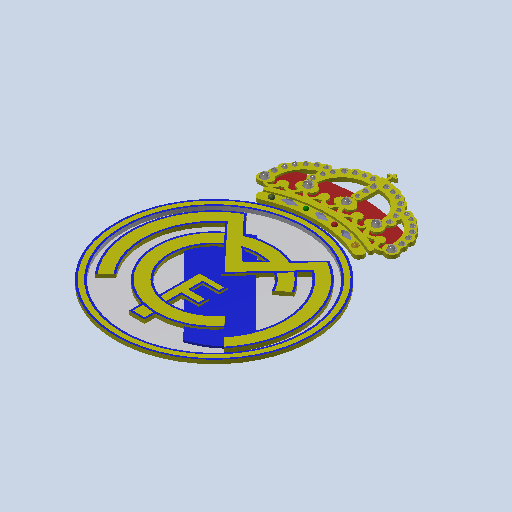
# Autodesk Inventor part: Part7
Saved by Autodesk Inventor 2024.2 (Build 282272000, 272)
## iProperties
Created: 2013-02-25
Part Number: Part7
Material: Generic
Document SubType Name: Modeling
Designer: bilal
Density: 1 g/cm^3
Appearance: Yellow
Author: bilal
Autodesk Inventor part; units mm, degrees
ref_plane "YZ Plane" through (0, 0, 0) normal (1, 0, 0) x (0, 1, 0)
ref_plane "XZ Plane" through (0, 0, 0) normal (0, 1, 0) x (-1, 0, 0)
ref_plane "XY Plane" through (0, 0, 0) normal (0, 0, 1) x (1, 0, 0)
sketch "Sketch1" plane through (0, 0, 0) normal (0, 0, 1) x (1, 0, 0)
  circle A0 centre (0, 0) radius 46.6203
  constraints: 1 centre point
extrude "Extrusion1" add sketch "Sketch1" along normal blind 1
sketch "Sketch2" plane through (0, 0, 1) normal (0, 0, 1) x (1, 0, 0)
  circle A0 centre (0, 0) radius 46.6203 projected
  circle A1 centre (0, 0) radius 51
  circle A2 centre (0, 0) radius 46.6203
  constraints: 2 centre point
extrude "Extrusion2" add sketch "Sketch2" along normal blind 2
sketch "Sketch3" plane through (0, 0, 1) normal (0, 0, 1) x (1, 0, 0)
  arc A0 (35.1776, -22.7841) -> (38.8842, -17.331) centre (7.3583, 0.1113) ccw
  line L0 (38.8842, -17.331) -> (-9.7309, 31.8301)
  arc A1 (-9.7309, 31.8301) -> (-26.8419, 11.4456) centre (7.3583, 0.1113) ccw
  line L1 (18.3098, -34.2133) -> (-26.8419, 11.4456)
  arc A2 (18.3098, -34.2133) -> (38.8842, -17.331) centre (7.3583, 0.1113) ccw
  line L2 (38.8842, -17.331) -> (11.8719, 9.9847)
  constraints: 6 end point, 6 point on circle, 3 centre point
extrude "Extrusion3" add sketch "Sketch3" along normal blind 1
sketch "Sketch4" plane through (0, 0, 1) normal (0, 0, 1) x (1, 0, 0)
  line L0 (7.1383, -0.1113) -> (-7.3583, -0.1113)
  line L1 (-7.3583, -0.1113) -> (-7.3583, -21.0954)
  arc A0 (-13.1155, 18.0871) -> (-7.3583, -21.0954) centre (0, 0) ccw
  line L2 (-13.1155, 18.0871) -> (-0.6206, 4.403)
  line L3 (-0.6206, 4.403) -> (12.5775, 18.4653)
  arc A1 (20.0006, 9.9568) -> (12.5775, 18.4653) centre (0, 0) ccw
  line L4 (20.0006, 9.9568) -> (26.5524, 15.0359)
  arc A2 (26.5524, 15.0359) -> (18.22, 24.4773) centre (0, 0) ccw
  line L5 (18.22, 24.4773) -> (22.0152, 28.521)
  arc A3 (27.8194, -22.8954) -> (22.0152, 28.521) centre (0, 0) ccw
  line L6 (27.8194, -22.8954) -> (33.5184, -28.2607)
  arc A4 (33.5184, -28.2607) -> (21.4165, 38.2555) centre (0, 0) ccw
  line L7 (21.4165, 38.2555) -> (11.8672, 28.1119)
  arc A5 (11.8672, 28.1119) -> (-11.8672, 28.1119) centre (0, 0) ccw
  line L8 (-11.8672, 28.1119) -> (-21.4067, 38.261)
  arc A6 (-21.4067, 38.261) -> (-33.3316, -28.4808) centre (0, 0) ccw
  line L9 (-33.3316, -28.4808) -> (-27.8194, -22.8954)
  arc A7 (-22.3813, 28.2346) -> (-27.8194, -22.8954) centre (0, 0) ccw
  line L10 (-22.3813, 28.2346) -> (-18.6516, 24.1501)
  arc A8 (-18.6516, 24.1501) -> (-8.045, -29.4345) centre (0, 0) ccw
  line L11 (-8.045, -29.4345) -> (-8.045, -36.0294)
  line L12 (-8.045, -36.0294) -> (0, -36.0294)
  line L13 (0, -36.0294) -> (0, -30.5141)
  arc A9 (0, -30.5141) -> (24.0395, -18.7939) centre (0, 0) ccw
  line L14 (24.0395, -18.7939) -> (18.3751, -12.7089)
  arc A10 (-1.6668, -22.2796) -> (18.3751, -12.7089) centre (0, 0) ccw
  line L15 (-1.6668, -22.2796) -> (-1.6668, -15.2832)
  line L16 (-1.6668, -15.2832) -> (7.3438, -15.2832)
  line L17 (7.3438, -15.2832) -> (7.3438, -10.1842)
  line L18 (7.3438, -10.1842) -> (-1.3429, -10.1842)
  line L19 (-1.3429, -10.1842) -> (-1.3429, -4.5649)
  line L20 (-1.3429, -4.5649) -> (7.1383, -4.5649)
  line L21 (7.1383, -4.5649) -> (7.1383, -0.1113)
  arc A11 (4.9662, 21.783) -> (-5.8652, 21.5583) centre (0, 0) ccw
  line L22 (-0.6206, 16.6817) -> (4.9662, 21.783)
  line L23 (-5.8652, 21.5583) -> (-0.6206, 16.6817)
  point P0 (0, 21.2286)
  constraints: 48 end point, 24 point on circle, 12 centre point
extrude "Extrusion4" add sketch "Sketch4" along normal blind 2
sketch "Sketch5" plane through (0, 0, 3) normal (0, 0, 1) x (1, 0, 0)
  arc A0 (-26.8477, 51.9535) -> (-24.7043, 47.4362) centre (-24.8696, 50.1249) ccw
  arc A1 (24.7043, 47.4362) -> (-24.7043, 47.4362) centre (0, -4.628) ccw
  arc A2 (24.7043, 47.4362) -> (26.8477, 51.9535) centre (24.6538, 50.2273) ccw
  arc A3 (26.8477, 51.9535) -> (-26.8477, 51.9535) centre (0, -4.628) ccw
  constraints: 8 point on circle, 4 centre point
extrude "Extrusion5" add sketch "Sketch5" against normal blind 2
sketch "Sketch6" plane through (0, 0, 3) normal (0, 0, 1) x (1, 0, 0)
  arc A0 (-21.8187, 53.0498) -> (-21.8187, 50.0443) centre (-21.8187, 51.5471) ccw
  line L0 (-21.8187, 53.0498) -> (-21.8187, 50.0443)
  point P0 (0, 0)
  constraints: 2 end point, 2 point on circle, 1 centre point, 1 midpoint, 1 vertical
revolve "Revolution1" add sketch "Sketch6" angle 180 about axis through (-21.8187, 53.0498, 3) along (0, 1, 0)
sketch "Sketch7" plane through (0, 0, 3) normal (0, 0, 1) x (1, 0, 0)
  arc A0 (-7.6781, 56.5711) -> (-7.6781, 54.1031) centre (-7.6781, 55.3371) ccw
  line L0 (-7.6781, 56.5711) -> (-7.6781, 54.1031)
  point P0 (0, 0)
  constraints: 2 end point, 2 point on circle, 1 centre point, 1 midpoint, 1 vertical
revolve "Revolution2" add sketch "Sketch7" angle 180 about axis through (-7.6781, 56.5711, 3) along (0, 1, 0)
sketch "Sketch8" plane through (0, 0, 3) normal (0, 0, 1) x (1, 0, 0)
  arc A0 (6.7914, 54.1951) -> (6.7914, 56.9016) centre (6.7914, 55.5484) ccw
  line L0 (6.7914, 56.9016) -> (6.7914, 54.1951)
  point P0 (0, 0)
  constraints: 2 end point, 2 point on circle, 1 centre point, 1 midpoint, 1 vertical
revolve "Revolution3" add sketch "Sketch8" angle 180 about axis through (6.7914, 56.9016, 3) along (0, -1, 0)
sketch "Sketch9" plane through (0, 0, 3) normal (0, 0, 1) x (1, 0, 0)
  arc A0 (21.5023, 49.9344) -> (21.5023, 53.17) centre (21.5023, 51.5522) ccw
  line L0 (21.5023, 53.17) -> (21.5023, 49.9344)
  point P0 (0, 0)
  constraints: 2 end point, 2 point on circle, 1 centre point, 1 midpoint, 1 vertical
revolve "Revolution4" add sketch "Sketch9" angle 180 about axis through (21.5023, 53.17, 3) along (0, -1, 0)
sketch "Sketch10" plane through (0, 0, 3) normal (0, 0, 1) x (1, 0, 0)
  line L0 (-14.6576, 52.3863) -> (-11.2239, 54.6397)
  line L1 (-11.2239, 54.6397) -> (-14.9744, 55.5777)
  line L2 (-14.9744, 55.5777) -> (-18.5205, 53.1374)
  line L3 (-18.5205, 53.1374) -> (-14.6576, 52.3863)
  point P0 (0, 0)
  constraints: 8 end point
extrude "Extrusion6" add sketch "Sketch10" along normal blind 1.353 draft -33
sketch "Sketch11" plane through (0, 0, 3) normal (0, 0, 1) x (1, 0, 0)
  line L0 (-3.7928, 55.8502) -> (-0.4654, 54.1271)
  line L1 (-0.1683, 57.514) -> (-3.7928, 55.8502)
  line L2 (-0.4654, 54.1271) -> (3.6345, 55.7908)
  line L3 (3.6345, 55.7908) -> (-0.1683, 57.514)
  point P0 (0, 0)
  constraints: 8 end point
extrude "Extrusion7" add sketch "Sketch11" along normal blind 1.353 draft -33
sketch "Sketch12" plane through (0, 0, 3) normal (0, 0, 1) x (1, 0, 0)
  line L0 (10.7052, 54.8996) -> (13.8544, 52.4634)
  line L1 (14.7456, 55.672) -> (10.7052, 54.8996)
  line L2 (18.1325, 52.9982) -> (14.7456, 55.672)
  line L3 (13.8544, 52.4634) -> (18.1325, 52.9982)
  point P0 (0, 0)
  constraints: 8 end point
extrude "Extrusion8" add sketch "Sketch12" along normal blind 1.353 draft -33
sketch "Sketch13" plane through (0, 0, 3) normal (0, 0, 1) x (1, 0, 0)
  arc A0 (27.2764, 52.857) -> (27.3948, 55.5395) centre (26.507, 54.2348) ccw
  arc A1 (27.3948, 55.5395) -> (31.0725, 56.5693) centre (28.3443, 59.2304) ccw
  arc A2 (31.0725, 56.5693) -> (34.8669, 61.608) centre (32.8513, 59.1778) ccw
  arc A3 (34.8669, 63.7336) -> (34.8669, 61.608) centre (37.3316, 62.6708) ccw
  arc A4 (34.8669, 63.7336) -> (34.3553, 65.7845) centre (32.9287, 64.3393) ccw
  arc A5 (34.2001, 67.4983) -> (34.3553, 65.7845) centre (35.5796, 66.7592) ccw
  arc A6 (34.2001, 67.4983) -> (32.9287, 71.112) centre (31.9885, 68.7507) ccw
  arc A7 (32.1807, 72.3878) -> (32.9287, 71.112) centre (33.4103, 72.2515) ccw
  arc A8 (32.1807, 72.3878) -> (30.8981, 74.2201) centre (30.2307, 72.3878) ccw
  arc A9 (29.6913, 75.332) -> (30.8981, 74.2201) centre (31.3651, 75.9379) ccw
  arc A10 (29.6913, 75.332) -> (27.6124, 77.2947) centre (27.6124, 75.2124) ccw
  arc A11 (26.3543, 78.0988) -> (27.6124, 77.2947) centre (28.1101, 79.4597) ccw
  arc A12 (26.3543, 78.0988) -> (23.8587, 79.736) centre (24.3371, 77.7446) ccw
  arc A13 (22.289, 80.8148) -> (23.8587, 79.736) centre (26.514, 85.2809) ccw
  arc A14 (22.289, 80.8148) -> (18.8818, 80.2204) centre (20.8447, 79.0315) ccw
  arc A15 (18.8818, 80.2204) -> (17.9847, 80.9244) centre (17.0645, 78.8282) ccw
  arc A16 (17.0204, 82.0412) -> (17.9847, 80.9244) centre (18.8265, 82.6261) ccw
  arc A17 (17.0204, 82.0412) -> (14.0111, 84.5648) centre (14.4576, 82.0412) ccw
  arc A18 (13.1122, 85.324) -> (14.0111, 84.5648) centre (14.4642, 86.0131) ccw
  arc A19 (13.1122, 85.324) -> (10.873, 86.717) centre (10.873, 84.2208) ccw
  arc A20 (9.707, 87.1556) -> (10.873, 86.717) centre (10.7721, 88.2181) ccw
  arc A21 (9.707, 87.1556) -> (6.892, 88.2551) centre (7.3694, 85.324) ccw
  arc A22 (5.0156, 88.4594) -> (6.892, 88.2551) centre (6.329, 91.8036) ccw
  arc A23 (5.0156, 88.4594) -> (2.066, 88.5941) centre (3.4226, 85.9398) ccw
  line L0 (2.066, 88.5941) -> (2.066, 89.3424)
  line L1 (2.066, 89.3424) -> (0.4888, 89.3424)
  line L2 (0.4888, 89.3424) -> (0.4888, 92.0213)
  line L3 (0.4888, 92.0213) -> (2.1357, 92.0213)
  line L4 (2.1357, 92.0213) -> (2.1357, 93.0772)
  line L5 (2.1357, 93.0772) -> (0.4888, 93.0772)
  line L6 (0.4888, 93.0772) -> (0.4888, 94.3608)
  line L7 (0.4888, 94.3608) -> (-0.6178, 94.3608)
  line L8 (-0.6178, 93.0772) -> (-0.6178, 94.3608)
  line L9 (-2.2647, 93.0772) -> (-0.6178, 93.0772)
  line L10 (-2.2647, 92.0213) -> (-2.2647, 93.0772)
  line L11 (-0.6178, 92.0213) -> (-2.2647, 92.0213)
  line L12 (-0.6178, 89.3424) -> (-0.6178, 92.0213)
  line L13 (-2.3707, 89.3424) -> (-0.6178, 89.3424)
  line L14 (-2.3707, 88.5974) -> (-2.3707, 89.3424)
  arc A24 (-2.3707, 88.5974) -> (-5.6472, 87.9561) centre (-3.5516, 85.9398) ccw
  arc A25 (-6.4012, 87.8566) -> (-5.6472, 87.9561) centre (-6.2139, 89.3436) ccw
  arc A26 (-6.4012, 87.8566) -> (-9.302, 87.4131) centre (-7.4983, 85.324) ccw
  arc A27 (-10.4406, 86.7726) -> (-9.302, 87.4131) centre (-11.9866, 90.8533) ccw
  arc A28 (-10.4406, 86.7726) -> (-13.3704, 85.324) centre (-11.0019, 84.2208) ccw
  arc A29 (-14.5865, 84.5332) -> (-13.3704, 85.324) centre (-14.3699, 85.5306) ccw
  arc A30 (-14.5865, 84.5332) -> (-16.9822, 82.7274) centre (-14.5865, 82.0412) ccw
  arc A31 (-17.6876, 81.0635) -> (-16.9822, 82.7274) centre (-21.8578, 83.8128) ccw
  arc A32 (-17.6876, 81.0635) -> (-19.0108, 80.2204) centre (-17.1934, 78.8282) ccw
  arc A33 (-19.0108, 80.2204) -> (-22.418, 80.8148) centre (-20.9736, 79.0315) ccw
  arc A34 (-23.9876, 79.736) -> (-22.418, 80.8148) centre (-26.643, 85.2809) ccw
  arc A35 (-23.9876, 79.736) -> (-26.4832, 78.0988) centre (-24.466, 77.7446) ccw
  arc A36 (-27.7413, 77.2947) -> (-26.4832, 78.0988) centre (-28.2391, 79.4597) ccw
  arc A37 (-27.7413, 77.2947) -> (-29.8202, 75.332) centre (-27.7413, 75.2124) ccw
  arc A38 (-31.027, 74.2201) -> (-29.8202, 75.332) centre (-31.4941, 75.9379) ccw
  arc A39 (-31.027, 74.2201) -> (-32.3097, 72.3878) centre (-30.3597, 72.3878) ccw
  arc A40 (-33.0577, 71.112) -> (-32.3097, 72.3878) centre (-33.5392, 72.2515) ccw
  arc A41 (-33.0577, 71.112) -> (-34.3291, 67.4983) centre (-32.1174, 68.7507) ccw
  arc A42 (-34.4842, 65.7845) -> (-34.3291, 67.4983) centre (-35.7085, 66.7592) ccw
  arc A43 (-34.4842, 65.7845) -> (-34.9959, 63.7336) centre (-33.0577, 64.3393) ccw
  arc A44 (-34.9959, 61.608) -> (-34.9959, 63.7336) centre (-37.4606, 62.6708) ccw
  arc A45 (-34.9959, 61.608) -> (-31.2014, 56.5693) centre (-32.9802, 59.1778) ccw
  arc A46 (-31.2014, 56.5693) -> (-27.2786, 55.6114) centre (-28.4733, 59.2304) ccw
  arc A47 (-27.2786, 55.6114) -> (-27.2764, 52.857) centre (-26.7799, 54.2346) ccw
  arc A48 (27.2764, 52.857) -> (-27.2764, 52.857) centre (0, -4.628) ccw
  arc A49 (-26.0136, 56.3094) -> (-24.6426, 59.0129) centre (-35.6939, 62.9182) ccw
  arc A50 (-24.6426, 59.0129) -> (-23.3101, 59.2794) centre (-24.1153, 59.8411) ccw
  arc A51 (-23.3101, 59.2794) -> (-20.9448, 58.2972) centre (-20.4128, 62.9176) ccw
  line L15 (-26.0136, 56.3094) -> (-20.9448, 58.2972)
  arc A52 (-18.4601, 59.2911) -> (-17.1363, 62.5661) centre (-21.1825, 62.2965) ccw
  arc A53 (-17.1363, 62.5661) -> (-16.4257, 62.6549) centre (-16.7931, 62.7074) ccw
  arc A54 (-16.4257, 62.6549) -> (-13.9877, 60.285) centre (-12.0514, 64.7157) ccw
  line L16 (-18.4601, 59.2911) -> (-13.9877, 60.285)
  arc A55 (-11.0061, 61.2788) -> (-9.2639, 63.034) centre (-13.5712, 65.5673) ccw
  arc A56 (-9.2639, 63.034) -> (-7.5609, 63.2438) centre (-8.5734, 64.4461) ccw
  arc A57 (-7.5609, 63.2438) -> (-5.99, 61.6262) centre (-5.2448, 63.9213) ccw
  line L17 (-11.0061, 61.2788) -> (-5.99, 61.6262)
  arc A58 (-2.6411, 61.8149) -> (-0.5696, 64.8302) centre (-5.2326, 65.8145) ccw
  arc A59 (-0.5696, 64.8302) -> (0.1176, 64.8305) centre (-0.2261, 65.0545) ccw
  arc A60 (0.1176, 64.8305) -> (1.7455, 61.9092) centre (4.7517, 65.4986) ccw
  line L18 (-2.6411, 61.8149) -> (1.7455, 61.9092)
  arc A61 (5.4311, 61.4871) -> (7.2144, 63.2692) centre (1.9408, 66.7629) ccw
  arc A62 (7.2144, 63.2692) -> (8.6844, 63.2278) centre (7.9871, 64.5875) ccw
  arc A63 (8.6844, 63.2278) -> (10.1889, 61.1777) centre (11.7929, 63.9318) ccw
  line L19 (5.4311, 61.4871) -> (10.1889, 61.1777)
  arc A64 (13.3984, 60.2835) -> (16.1185, 62.6849) centre (10.7455, 66.0297) ccw
  arc A65 (16.1185, 62.6849) -> (16.8326, 62.2884) centre (16.5732, 62.6625) ccw
  arc A66 (16.8326, 62.2884) -> (17.5857, 59.3699) centre (20.4564, 61.6671) ccw
  line L20 (13.3984, 60.2835) -> (17.5857, 59.3699)
  arc A67 (20.7071, 58.4563) -> (23.4267, 59.3699) centre (19.5919, 66.2806) ccw
  arc A68 (23.4267, 59.3699) -> (24.4767, 59.0763) centre (24.0109, 59.435) ccw
  arc A69 (24.4767, 59.0763) -> (25.3892, 56.4769) centre (36.9067, 61.9797) ccw
  line L21 (20.7071, 58.4563) -> (25.3892, 56.4769)
  arc A70 (-30.1852, 57.1125) -> (-26.8854, 58.9221) centre (-29.0998, 59.0467) ccw
  arc A71 (-30.1852, 57.1125) -> (-30.2916, 61.6897) centre (-31.2887, 59.3767) ccw
  arc A72 (-21.4566, 75.6341) -> (-30.2916, 61.6897) centre (-16.1684, 62.5124) ccw
  arc A73 (-21.4566, 75.6341) -> (-21.0309, 73.2923) centre (-9.925, 76.5211) ccw
  arc A74 (-21.0309, 73.2923) -> (-20.818, 69.1409) centre (-20.4492, 71.241) ccw
  line L22 (-21.0309, 67.4378) -> (-20.818, 69.1409)
  arc A75 (-21.0309, 67.4378) -> (-18.5826, 62.5413) centre (-19.3005, 65.2427) ccw
  arc A76 (-22.734, 60.9446) -> (-18.5826, 62.5413) centre (-20.9295, 62.4481) ccw
  arc A77 (-22.734, 60.9446) -> (-26.8854, 58.9221) centre (-25.1398, 60.611) ccw
  arc A78 (26.7564, 58.9221) -> (30.0562, 57.1125) centre (28.9708, 59.0467) ccw
  arc A79 (26.7564, 58.9221) -> (22.605, 60.9446) centre (25.0108, 60.611) ccw
  arc A80 (18.4537, 62.5413) -> (22.605, 60.9446) centre (20.8006, 62.4481) ccw
  arc A81 (18.4537, 62.5413) -> (20.9019, 67.4378) centre (19.1715, 65.2427) ccw
  line L23 (20.689, 69.1409) -> (20.9019, 67.4378)
  arc A82 (20.689, 69.1409) -> (20.9019, 73.2923) centre (20.3202, 71.241) ccw
  arc A83 (20.9019, 73.2923) -> (21.3277, 75.6341) centre (9.7961, 76.5211) ccw
  arc A84 (30.1627, 61.6897) -> (21.3277, 75.6341) centre (16.0394, 62.5124) ccw
  arc A85 (30.1627, 61.6897) -> (30.0562, 57.1125) centre (31.1597, 59.3767) ccw
  arc A86 (-14.85, 63.3928) -> (-12.721, 61.6897) centre (-12.9146, 63.6299) ccw
  arc A87 (-14.85, 63.3928) -> (-15.1693, 68.8216) centre (-15.4757, 66.0798) ccw
  arc A88 (-15.1693, 68.8216) -> (-16.8724, 69.9925) centre (-17.1409, 67.7779) ccw
  arc A89 (-2.2894, 82.9789) -> (-16.8724, 69.9925) centre (-2.6896, 68.747) ccw
  line L24 (-2.2894, 74.0267) -> (-2.2894, 82.9789)
  arc A90 (-2.2894, 74.0267) -> (-0.8638, 72.6103) centre (-1.15, 73.7478) ccw
  line L25 (-0.8638, 72.2357) -> (-0.8638, 72.6103)
  arc A91 (-0.8638, 72.2357) -> (-3.3538, 70.5247) centre (-1.1343, 69.962) ccw
  arc A92 (-3.3538, 70.5247) -> (-1.8636, 65.6282) centre (-2.6852, 68.0532) ccw
  arc A93 (-3.7796, 62.9671) -> (-1.8636, 65.6282) centre (-4.7945, 65.7181) ccw
  arc A94 (-6.5472, 64.4573) -> (-3.7796, 62.9671) centre (-3.1651, 67.4233) ccw
  arc A95 (-6.5472, 64.4573) -> (-10.5921, 64.2444) centre (-8.6357, 65.6052) ccw
  arc A96 (-12.721, 61.6897) -> (-10.5921, 64.2444) centre (-13.4498, 64.4614) ccw
  arc A97 (15.0403, 68.8216) -> (14.721, 63.3928) centre (15.3468, 66.0798) ccw
  arc A98 (12.5921, 61.6897) -> (14.721, 63.3928) centre (12.7856, 63.6299) ccw
  arc A99 (10.4632, 64.2444) -> (12.5921, 61.6897) centre (13.3208, 64.4614) ccw
  arc A100 (10.4632, 64.2444) -> (6.4182, 64.4573) centre (8.5067, 65.6052) ccw
  arc A101 (3.6507, 62.9671) -> (6.4182, 64.4573) centre (3.0362, 67.4233) ccw
  arc A102 (1.7346, 65.6282) -> (3.6507, 62.9671) centre (4.6656, 65.7181) ccw
  arc A103 (1.7346, 65.6282) -> (3.2249, 70.5247) centre (2.4032, 68.0997) ccw
  arc A104 (3.2249, 70.5247) -> (0.7348, 72.2357) centre (1.0054, 69.962) ccw
  line L26 (0.7348, 72.6103) -> (0.7348, 72.2357)
  arc A105 (0.7348, 72.6103) -> (2.1604, 74.0267) centre (1.0211, 73.7478) ccw
  line L27 (2.1604, 82.9789) -> (2.1604, 74.0267)
  arc A106 (16.7435, 69.9925) -> (2.1604, 82.9789) centre (2.5606, 68.747) ccw
  arc A107 (16.7435, 69.9925) -> (15.0403, 68.8216) centre (17.0119, 67.7779) ccw
  point P0 (0, 0)
  constraints: 216 point on circle, 108 centre point, 56 end point
extrude "Extrusion9" add sketch "Sketch13" against normal blind 2
sketch "Sketch14" plane through (0, 0, 3) normal (0, 0, 1) x (1, 0, 0)
  line L0 (-2.3707, 88.5974) -> (-2.3707, 89.3424) projected
  arc A0 (-32.9802, 57.0588) -> (-32.9802, 61.2969) centre (-32.9802, 59.1778) ccw
  line L1 (-32.9802, 61.2969) -> (-32.9802, 57.0588)
  point P0 (0, 0)
  constraints: 2 end point, 2 point on circle, 1 centre point, 1 midpoint, 1 parallel
revolve "Revolution5" add sketch "Sketch14" angle 180 about axis through (-32.9802, 61.2969, 3) along (0, -1, 0)
sketch "Sketch15" plane through (0, 0, 3) normal (0, 0, 1) x (1, 0, 0)
  line L0 (-2.3707, 88.5974) -> (-2.3707, 89.3424) projected
  arc A0 (-33.0577, 63.0233) -> (-33.0577, 65.6553) centre (-33.0577, 64.3393) ccw
  line L1 (-33.0577, 65.6553) -> (-33.0577, 63.0233)
  point P0 (0, 0)
  constraints: 2 end point, 2 point on circle, 1 centre point, 1 midpoint, 1 parallel
revolve "Revolution6" add sketch "Sketch15" angle 180 about axis through (-33.0577, 65.6553, 3) along (0, -1, 0)
sketch "Sketch16" plane through (0, 0, 3) normal (0, 0, 1) x (1, 0, 0)
  line L0 (-2.3707, 88.5974) -> (-2.3707, 89.3424) projected
  arc A0 (-32.1174, 67.4278) -> (-32.1174, 70.0735) centre (-32.1174, 68.7507) ccw
  line L1 (-32.1174, 70.0735) -> (-32.1174, 67.4278)
  point P0 (0, 0)
  constraints: 2 end point, 2 point on circle, 1 centre point, 1 midpoint, 1 parallel
revolve "Revolution7" add sketch "Sketch16" angle 180 about axis through (-32.1174, 70.0735, 3) along (0, -1, 0)
sketch "Sketch17" plane through (0, 0, 3) normal (0, 0, 1) x (1, 0, 0)
  line L0 (-2.3707, 88.5974) -> (-2.3707, 89.3424) projected
  arc A0 (-30.3597, 71.1446) -> (-30.3597, 73.631) centre (-30.3597, 72.3878) ccw
  line L1 (-30.3597, 73.631) -> (-30.3597, 71.1446)
  point P0 (0, 0)
  constraints: 2 end point, 2 point on circle, 1 centre point, 1 midpoint, 1 parallel
revolve "Revolution8" add sketch "Sketch17" angle 180 about axis through (-30.3597, 73.631, 3) along (0, -1, 0)
sketch "Sketch18" plane through (0, 0, 3) normal (0, 0, 1) x (1, 0, 0)
  line L0 (-2.3707, 88.5974) -> (-2.3707, 89.3424) projected
  arc A0 (-27.7413, 74.0384) -> (-27.7413, 76.3864) centre (-27.7413, 75.2124) ccw
  line L1 (-27.7413, 76.3864) -> (-27.7413, 74.0384)
  point P0 (0, 0)
  constraints: 2 end point, 2 point on circle, 1 centre point, 1 midpoint, 1 parallel
revolve "Revolution9" add sketch "Sketch18" angle 180 about axis through (-27.7413, 76.3864, 3) along (0, -1, 0)
sketch "Sketch19" plane through (0, 0, 3) normal (0, 0, 1) x (1, 0, 0)
  line L0 (-2.3707, 88.5974) -> (-2.3707, 89.3424) projected
  arc A0 (-24.466, 76.6232) -> (-24.466, 78.8659) centre (-24.466, 77.7446) ccw
  line L1 (-24.466, 78.8659) -> (-24.466, 76.6232)
  point P0 (0, 0)
  constraints: 2 end point, 2 point on circle, 1 centre point, 1 midpoint, 1 parallel
revolve "Revolution10" add sketch "Sketch19" angle 180 about axis through (-24.466, 78.8659, 3) along (0, -1, 0)
sketch "Sketch20" plane through (0, 0, 3) normal (0, 0, 1) x (1, 0, 0)
  line L0 (-2.3707, 88.5974) -> (-2.3707, 89.3424) projected
  arc A0 (-20.9736, 77.9173) -> (-20.9736, 80.1457) centre (-20.9736, 79.0315) ccw
  line L1 (-20.9736, 80.1457) -> (-20.9736, 77.9173)
  point P0 (0, 0)
  constraints: 2 end point, 2 point on circle, 1 centre point, 1 midpoint, 1 parallel
revolve "Revolution11" add sketch "Sketch20" angle 180 about axis through (-20.9736, 80.1457, 3) along (0, -1, 0)
sketch "Sketch21" plane through (0, 0, 3) normal (0, 0, 1) x (1, 0, 0)
  line L0 (-2.3707, 88.5974) -> (-2.3707, 89.3424) projected
  arc A0 (-17.6876, 64.2364) -> (-17.6876, 68.709) centre (-17.6876, 66.4727) ccw
  line L1 (-17.6876, 68.709) -> (-17.6876, 64.2364)
  point P0 (0, 0)
  constraints: 2 end point, 2 point on circle, 1 centre point, 1 midpoint, 1 parallel
revolve "Revolution12" add sketch "Sketch21" angle 180 about axis through (-17.6876, 68.709, 3) along (0, -1, 0)
sketch "Sketch22" plane through (0, 0, 3) normal (0, 0, 1) x (1, 0, 0)
  line L0 (-2.3707, 88.5974) -> (-2.3707, 89.3424) projected
  arc A0 (-19.8735, 69.8473) -> (-19.8735, 72.3288) centre (-19.8735, 71.0881) ccw
  line L1 (-19.8735, 72.3288) -> (-19.8735, 69.8473)
  point P0 (0, 0)
  constraints: 2 end point, 2 point on circle, 1 centre point, 1 midpoint, 1 parallel
revolve "Revolution13" add sketch "Sketch22" angle 180 about axis through (-19.8735, 72.3288, 3) along (0, -1, 0)
sketch "Sketch23" plane through (0, 0, 3) normal (0, 0, 1) x (1, 0, 0)
  line L0 (-2.3707, 88.5974) -> (-2.3707, 89.3424) projected
  arc A0 (-18.9005, 74.1389) -> (-18.9005, 76.4685) centre (-18.9005, 75.3037) ccw
  line L1 (-18.9005, 76.4685) -> (-18.9005, 74.1389)
  point P0 (0, 0)
  constraints: 2 end point, 2 point on circle, 1 centre point, 1 midpoint, 1 parallel
revolve "Revolution14" add sketch "Sketch23" angle 180 about axis through (-18.9005, 76.4685, 3) along (0, -1, 0)
sketch "Sketch24" plane through (0, 0, 3) normal (0, 0, 1) x (1, 0, 0)
  line L0 (-2.3707, 88.5974) -> (-2.3707, 89.3424) projected
  arc A0 (-17.1934, 77.7383) -> (-17.1934, 79.918) centre (-17.1934, 78.8282) ccw
  line L1 (-17.1934, 79.918) -> (-17.1934, 77.7383)
  point P0 (0, 0)
  constraints: 2 end point, 2 point on circle, 1 centre point, 1 midpoint, 1 parallel
revolve "Revolution15" add sketch "Sketch24" angle 180 about axis through (-17.1934, 79.918, 3) along (0, -1, 0)
sketch "Sketch25" plane through (0, 0, 3) normal (0, 0, 1) x (1, 0, 0)
  line L0 (-2.3707, 88.5974) -> (-2.3707, 89.3424) projected
  arc A0 (-14.5865, 80.776) -> (-14.5865, 83.3064) centre (-14.5865, 82.0412) ccw
  line L1 (-14.5865, 83.3064) -> (-14.5865, 80.776)
  point P0 (0, 0)
  constraints: 2 end point, 2 point on circle, 1 centre point, 1 midpoint, 1 parallel
revolve "Revolution16" add sketch "Sketch25" angle 180 about axis through (-14.5865, 83.3064, 3) along (0, -1, 0)
sketch "Sketch26" plane through (0, 0, 3) normal (0, 0, 1) x (1, 0, 0)
  line L0 (-2.3707, 88.5974) -> (-2.3707, 89.3424) projected
  arc A0 (-11.0019, 83.0375) -> (-11.0019, 85.4042) centre (-11.0019, 84.2208) ccw
  line L1 (-11.0019, 85.4042) -> (-11.0019, 83.0375)
  point P0 (0, 0)
  constraints: 2 end point, 2 point on circle, 1 centre point, 1 midpoint, 1 parallel
revolve "Revolution17" add sketch "Sketch26" angle 180 about axis through (-11.0019, 85.4042, 3) along (0, -1, 0)
sketch "Sketch27" plane through (0, 0, 3) normal (0, 0, 1) x (1, 0, 0)
  line L0 (-2.3707, 88.5974) -> (-2.3707, 89.3424) projected
  arc A0 (-7.4983, 84.2055) -> (-7.4983, 86.4424) centre (-7.4983, 85.324) ccw
  line L1 (-7.4983, 86.4424) -> (-7.4983, 84.2055)
  point P0 (0, 0)
  constraints: 2 end point, 2 point on circle, 1 centre point, 1 midpoint, 1 parallel
revolve "Revolution18" add sketch "Sketch27" angle 180 about axis through (-7.4983, 86.4424, 3) along (0, -1, 0)
sketch "Sketch28" plane through (0, 0, 3) normal (0, 0, 1) x (1, 0, 0)
  line L0 (-2.3707, 88.5974) -> (-2.3707, 89.3424) projected
  arc A0 (-3.5516, 84.6849) -> (-3.5516, 87.1946) centre (-3.5516, 85.9398) ccw
  line L1 (-3.5516, 87.1946) -> (-3.5516, 84.6849)
  point P0 (0, 0)
  constraints: 2 end point, 2 point on circle, 1 centre point, 1 midpoint, 1 parallel
revolve "Revolution19" add sketch "Sketch28" angle 180 about axis through (-3.5516, 87.1946, 3) along (0, -1, 0)
sketch "Sketch29" plane through (0, 0, 3) normal (0, 0, 1) x (1, 0, 0)
  line L0 (-2.3707, 88.5974) -> (-2.3707, 89.3424) projected
  arc A0 (-0.1053, 81.3935) -> (-0.1053, 84.0612) centre (-0.1053, 82.7274) ccw
  line L1 (-0.1053, 84.0612) -> (-0.1053, 81.3935)
  point P0 (0, 0)
  constraints: 2 end point, 2 point on circle, 1 centre point, 1 midpoint, 1 parallel
revolve "Revolution20" add sketch "Sketch29" angle 180 about axis through (-0.1053, 84.0612, 3) along (0, -1, 0)
sketch "Sketch30" plane through (0, 0, 3) normal (0, 0, 1) x (1, 0, 0)
  line L0 (-2.3707, 88.5974) -> (-2.3707, 89.3424) projected
  arc A0 (-0.1143, 77.4016) -> (-0.1143, 79.9183) centre (-0.1143, 78.6599) ccw
  line L1 (-0.1143, 79.9183) -> (-0.1143, 77.4016)
  point P0 (0, 0)
  constraints: 2 end point, 2 point on circle, 1 centre point, 1 midpoint, 1 parallel
revolve "Revolution21" add sketch "Sketch30" angle 180 about axis through (-0.1143, 79.9183, 3) along (0, -1, 0)
sketch "Sketch31" plane through (0, 0, 3) normal (0, 0, 1) x (1, 0, 0)
  line L0 (-2.3707, 88.5974) -> (-2.3707, 89.3424) projected
  arc A0 (-0.0392, 73.4035) -> (-0.0392, 75.4545) centre (-0.0392, 74.429) ccw
  line L1 (-0.0392, 75.4545) -> (-0.0392, 73.4035)
  point P0 (0, 0)
  constraints: 2 end point, 2 point on circle, 1 centre point, 1 midpoint, 1 parallel
revolve "Revolution22" add sketch "Sketch31" angle 180 about axis through (-0.0392, 75.4545, 3) along (0, -1, 0)
sketch "Sketch32" plane through (0, 0, 3) normal (0, 0, 1) x (1, 0, 0)
  line L0 (-2.3707, 88.5974) -> (-2.3707, 89.3424) projected
  arc A0 (-0.2879, 66.7067) -> (-0.2879, 70.8389) centre (-0.2879, 68.7728) ccw
  line L1 (-0.2879, 70.8389) -> (-0.2879, 66.7067)
  point P0 (0, 0)
  dimension "d3" = 0
  constraints: 2 end point, 2 point on circle, 1 centre point, 1 midpoint, 1 parallel
revolve "Revolution23" add sketch "Sketch32" angle 180 about axis through (-0.2879, 70.8389, 3) along (0, -1, 0)
sketch "Sketch33" plane through (0, 0, 3) normal (0, 0, 1) x (1, 0, 0)
  line L0 (-2.3707, 88.5974) -> (-2.3707, 89.3424) projected
  arc A0 (3.4226, 84.6849) -> (3.4226, 87.1946) centre (3.4226, 85.9398) ccw
  line L1 (3.4226, 87.1946) -> (3.4226, 84.6849)
  point P0 (0, 0)
  constraints: 2 end point, 2 point on circle, 1 centre point, 1 midpoint, 1 parallel
revolve "Revolution24" add sketch "Sketch33" angle 180 about axis through (3.4226, 87.1946, 3) along (0, -1, 0)
sketch "Sketch34" plane through (0, 0, 3) normal (0, 0, 1) x (1, 0, 0)
  line L0 (-2.3707, 88.5974) -> (-2.3707, 89.3424) projected
  arc A0 (7.3694, 84.2055) -> (7.3694, 86.4424) centre (7.3694, 85.324) ccw
  line L1 (7.3694, 86.4424) -> (7.3694, 84.2055)
  point P0 (0, 0)
  constraints: 2 end point, 2 point on circle, 1 centre point, 1 midpoint, 1 parallel
revolve "Revolution25" add sketch "Sketch34" angle 180 about axis through (7.3694, 86.4424, 3) along (0, -1, 0)
sketch "Sketch35" plane through (0, 0, 3) normal (0, 0, 1) x (1, 0, 0)
  line L0 (-2.3707, 88.5974) -> (-2.3707, 89.3424) projected
  arc A0 (10.873, 83.0375) -> (10.873, 85.4042) centre (10.873, 84.2208) ccw
  line L1 (10.873, 85.4042) -> (10.873, 83.0375)
  point P0 (0, 0)
  constraints: 2 end point, 2 point on circle, 1 centre point, 1 midpoint, 1 parallel
revolve "Revolution26" add sketch "Sketch35" angle 180 about axis through (10.873, 85.4042, 3) along (0, -1, 0)
sketch "Sketch36" plane through (0, 0, 3) normal (0, 0, 1) x (1, 0, 0)
  line L0 (-2.3707, 88.5974) -> (-2.3707, 89.3424) projected
  arc A0 (14.4576, 80.776) -> (14.4576, 83.3064) centre (14.4576, 82.0412) ccw
  line L1 (14.4576, 83.3064) -> (14.4576, 80.776)
  point P0 (0, 0)
  constraints: 2 end point, 2 point on circle, 1 centre point, 1 midpoint, 1 parallel
revolve "Revolution27" add sketch "Sketch36" angle 180 about axis through (14.4576, 83.3064, 3) along (0, -1, 0)
sketch "Sketch37" plane through (0, 0, 3) normal (0, 0, 1) x (1, 0, 0)
  line L0 (-2.3707, 88.5974) -> (-2.3707, 89.3424) projected
  arc A0 (17.0645, 77.7383) -> (17.0645, 79.918) centre (17.0645, 78.8282) ccw
  line L1 (17.0645, 79.918) -> (17.0645, 77.7383)
  point P0 (0, 0)
  constraints: 2 end point, 2 point on circle, 1 centre point, 1 midpoint, 1 parallel
revolve "Revolution28" add sketch "Sketch37" angle 180 about axis through (17.0645, 79.918, 3) along (0, -1, 0)
sketch "Sketch38" plane through (0, 0, 3) normal (0, 0, 1) x (1, 0, 0)
  line L0 (-2.3707, 88.5974) -> (-2.3707, 89.3424) projected
  arc A0 (20.8447, 77.9173) -> (20.8447, 80.1457) centre (20.8447, 79.0315) ccw
  line L1 (20.8447, 80.1457) -> (20.8447, 77.9173)
  point P0 (0, 0)
  constraints: 2 end point, 2 point on circle, 1 centre point, 1 midpoint, 1 parallel
revolve "Revolution29" add sketch "Sketch38" angle 180 about axis through (20.8447, 80.1457, 3) along (0, -1, 0)
sketch "Sketch39" plane through (0, 0, 3) normal (0, 0, 1) x (1, 0, 0)
  line L0 (-2.3707, 88.5974) -> (-2.3707, 89.3424) projected
  arc A0 (24.3371, 76.6232) -> (24.3371, 78.8659) centre (24.3371, 77.7446) ccw
  line L1 (24.3371, 78.8659) -> (24.3371, 76.6232)
  point P0 (0, 0)
  constraints: 2 end point, 2 point on circle, 1 centre point, 1 midpoint, 1 parallel
revolve "Revolution30" add sketch "Sketch39" angle 180 about axis through (24.3371, 78.8659, 3) along (0, -1, 0)
sketch "Sketch40" plane through (0, 0, 3) normal (0, 0, 1) x (1, 0, 0)
  line L0 (-2.3707, 88.5974) -> (-2.3707, 89.3424) projected
  arc A0 (18.7715, 74.1389) -> (18.7715, 76.4685) centre (18.7715, 75.3037) ccw
  line L1 (18.7715, 76.4685) -> (18.7715, 74.1389)
  point P0 (0, 0)
  constraints: 2 end point, 2 point on circle, 1 centre point, 1 midpoint, 1 parallel
revolve "Revolution31" add sketch "Sketch40" angle 180 about axis through (18.7715, 76.4685, 3) along (0, -1, 0)
sketch "Sketch41" plane through (0, 0, 3) normal (0, 0, 1) x (1, 0, 0)
  line L0 (-2.3707, 88.5974) -> (-2.3707, 89.3424) projected
  arc A0 (19.7446, 69.8473) -> (19.7446, 72.3288) centre (19.7446, 71.0881) ccw
  line L1 (19.7446, 72.3288) -> (19.7446, 69.8473)
  point P0 (0, 0)
  constraints: 2 end point, 2 point on circle, 1 centre point, 1 midpoint, 1 parallel
revolve "Revolution32" add sketch "Sketch41" angle 180 about axis through (19.7446, 72.3288, 3) along (0, -1, 0)
sketch "Sketch42" plane through (0, 0, 3) normal (0, 0, 1) x (1, 0, 0)
  line L0 (-2.3707, 88.5974) -> (-2.3707, 89.3424) projected
  arc A0 (17.5586, 64.2364) -> (17.5586, 68.709) centre (17.5586, 66.4727) ccw
  line L1 (17.5586, 68.709) -> (17.5586, 64.2364)
  point P0 (0, 0)
  constraints: 2 end point, 2 point on circle, 1 centre point, 1 midpoint, 1 parallel
revolve "Revolution33" add sketch "Sketch42" angle 180 about axis through (17.5586, 68.709, 3) along (0, -1, 0)
sketch "Sketch43" plane through (0, 0, 3) normal (0, 0, 1) x (1, 0, 0)
  line L0 (-2.3707, 88.5974) -> (-2.3707, 89.3424) projected
  arc A0 (27.6124, 74.0384) -> (27.6124, 76.3864) centre (27.6124, 75.2124) ccw
  line L1 (27.6124, 76.3864) -> (27.6124, 74.0384)
  point P0 (0, 0)
  constraints: 2 end point, 2 point on circle, 1 centre point, 1 midpoint, 1 parallel
revolve "Revolution34" add sketch "Sketch43" angle 180 about axis through (27.6124, 76.3864, 3) along (0, -1, 0)
sketch "Sketch44" plane through (0, 0, 3) normal (0, 0, 1) x (1, 0, 0)
  line L0 (-2.3707, 88.5974) -> (-2.3707, 89.3424) projected
  arc A0 (30.2307, 71.1446) -> (30.2307, 73.631) centre (30.2307, 72.3878) ccw
  line L1 (30.2307, 73.631) -> (30.2307, 71.1446)
  point P0 (0, 0)
  constraints: 2 end point, 2 point on circle, 1 centre point, 1 midpoint, 1 parallel
revolve "Revolution35" add sketch "Sketch44" angle 180 about axis through (30.2307, 73.631, 3) along (0, -1, 0)
sketch "Sketch45" plane through (0, 0, 3) normal (0, 0, 1) x (1, 0, 0)
  line L0 (-2.3707, 88.5974) -> (-2.3707, 89.3424) projected
  arc A0 (31.9885, 67.4278) -> (31.9885, 70.0735) centre (31.9885, 68.7507) ccw
  line L1 (31.9885, 70.0735) -> (31.9885, 67.4278)
  point P0 (0, 0)
  constraints: 2 end point, 2 point on circle, 1 centre point, 1 midpoint, 1 parallel
revolve "Revolution36" add sketch "Sketch45" angle 180 about axis through (31.9885, 70.0735, 3) along (0, -1, 0)
sketch "Sketch46" plane through (0, 0, 3) normal (0, 0, 1) x (1, 0, 0)
  line L0 (-2.3707, 88.5974) -> (-2.3707, 89.3424) projected
  arc A0 (32.9287, 63.0233) -> (32.9287, 65.6553) centre (32.9287, 64.3393) ccw
  line L1 (32.9287, 65.6553) -> (32.9287, 63.0233)
  point P0 (0, 0)
  constraints: 2 end point, 2 point on circle, 1 centre point, 1 midpoint, 1 parallel
revolve "Revolution37" add sketch "Sketch46" angle 180 about axis through (32.9287, 65.6553, 3) along (0, -1, 0)
sketch "Sketch47" plane through (0, 0, 3) normal (0, 0, 1) x (1, 0, 0)
  line L0 (-2.3707, 88.5974) -> (-2.3707, 89.3424) projected
  arc A0 (32.8513, 57.0588) -> (32.8513, 61.2969) centre (32.8513, 59.1778) ccw
  line L1 (32.8513, 61.2969) -> (32.8513, 57.0588)
  point P0 (0, 0)
  constraints: 2 end point, 2 point on circle, 1 centre point, 1 midpoint, 1 parallel
revolve "Revolution38" add sketch "Sketch47" angle 180 about axis through (32.8513, 61.2969, 3) along (0, -1, 0)
sketch "Sketch49" plane through (0, 0, 1) normal (0, 0, -1) x (-1, 0, 0)
  arc A0 (-14.721, 63.3928) -> (-12.5921, 61.6897) centre (-12.7856, 63.6299) ccw projected
  arc A1 (-14.721, 63.3928) -> (-15.0403, 68.8216) centre (-15.3468, 66.0798) ccw projected
  arc A2 (-15.0403, 68.8216) -> (-16.7435, 69.9925) centre (-17.0119, 67.7779) ccw projected
  arc A3 (-2.1604, 82.9789) -> (-16.7435, 69.9925) centre (-2.5606, 68.747) ccw projected
  line L0 (-2.1604, 82.9789) -> (-2.1604, 74.0267) projected
  arc A4 (-2.1604, 74.0267) -> (-0.7348, 72.6103) centre (-1.0211, 73.7478) ccw projected
  line L1 (-0.7348, 72.6103) -> (-0.7348, 72.2357) projected
  arc A5 (-0.7348, 72.2357) -> (-3.2249, 70.5247) centre (-1.0054, 69.962) ccw projected
  arc A6 (-3.2249, 70.5247) -> (-1.7346, 65.6282) centre (-2.4032, 68.0997) ccw projected
  arc A7 (-3.6507, 62.9671) -> (-1.7346, 65.6282) centre (-4.6656, 65.7181) ccw projected
  arc A8 (-6.4182, 64.4573) -> (-3.6507, 62.9671) centre (-3.0362, 67.4233) ccw projected
  arc A9 (-6.4182, 64.4573) -> (-10.4632, 64.2444) centre (-8.5067, 65.6052) ccw projected
  arc A10 (-12.5921, 61.6897) -> (-10.4632, 64.2444) centre (-13.3208, 64.4614) ccw projected
  arc A11 (16.8724, 69.9925) -> (2.2894, 82.9789) centre (2.6896, 68.747) ccw projected
  arc A12 (16.8724, 69.9925) -> (15.1693, 68.8216) centre (17.1409, 67.7779) ccw projected
  arc A13 (15.1693, 68.8216) -> (14.85, 63.3928) centre (15.4757, 66.0798) ccw projected
  arc A14 (12.721, 61.6897) -> (14.85, 63.3928) centre (12.9146, 63.6299) ccw projected
  arc A15 (10.5921, 64.2444) -> (12.721, 61.6897) centre (13.4498, 64.4614) ccw projected
  arc A16 (10.5921, 64.2444) -> (6.5472, 64.4573) centre (8.6357, 65.6052) ccw projected
  arc A17 (3.7796, 62.9671) -> (6.5472, 64.4573) centre (3.1651, 67.4233) ccw projected
  arc A18 (1.8636, 65.6282) -> (3.7796, 62.9671) centre (4.7945, 65.7181) ccw projected
  arc A19 (1.8636, 65.6282) -> (3.3538, 70.5247) centre (2.6852, 68.0532) ccw projected
  arc A20 (3.3538, 70.5247) -> (0.8638, 72.2357) centre (1.1343, 69.962) ccw projected
  line L2 (0.8638, 72.2357) -> (0.8638, 72.6103) projected
  arc A21 (0.8638, 72.6103) -> (2.2894, 74.0267) centre (1.15, 73.7478) ccw projected
  line L3 (2.2894, 74.0267) -> (2.2894, 82.9789) projected
  arc A22 (-20.9019, 73.2923) -> (-20.689, 69.1409) centre (-20.3202, 71.241) ccw projected
  line L4 (-20.689, 69.1409) -> (-20.9019, 67.4378) projected
  arc A23 (-20.9019, 67.4378) -> (-18.4537, 62.5413) centre (-19.1715, 65.2427) ccw projected
  arc A24 (-22.605, 60.9446) -> (-18.4537, 62.5413) centre (-20.8006, 62.4481) ccw projected
  arc A25 (-22.605, 60.9446) -> (-26.7564, 58.9221) centre (-25.0108, 60.611) ccw projected
  arc A26 (-30.0562, 57.1125) -> (-26.7564, 58.9221) centre (-28.9708, 59.0467) ccw projected
  arc A27 (-30.0562, 57.1125) -> (-30.1627, 61.6897) centre (-31.1597, 59.3767) ccw projected
  arc A28 (-21.3277, 75.6341) -> (-30.1627, 61.6897) centre (-16.0394, 62.5124) ccw projected
  arc A29 (26.8854, 58.9221) -> (30.1852, 57.1125) centre (29.0998, 59.0467) ccw projected
  arc A30 (26.8854, 58.9221) -> (22.734, 60.9446) centre (25.1398, 60.611) ccw projected
  arc A31 (18.5826, 62.5413) -> (22.734, 60.9446) centre (20.9295, 62.4481) ccw projected
  arc A32 (18.5826, 62.5413) -> (21.0309, 67.4378) centre (19.3005, 65.2427) ccw projected
  line L5 (21.0309, 67.4378) -> (20.818, 69.1409) projected
  arc A33 (20.818, 69.1409) -> (21.0309, 73.2923) centre (20.4492, 71.241) ccw projected
  arc A34 (30.2916, 61.6897) -> (21.4566, 75.6341) centre (16.1684, 62.5124) ccw projected
  arc A35 (30.2916, 61.6897) -> (30.1852, 57.1125) centre (31.2887, 59.3767) ccw projected
  line L6 (2.6411, 61.8149) -> (-1.7455, 61.9092) projected
  arc A36 (-1.7455, 61.9092) -> (-0.1176, 64.8305) centre (-4.7517, 65.4986) ccw projected
  arc A37 (-0.1176, 64.8305) -> (0.5696, 64.8302) centre (0.2261, 65.0545) ccw projected
  arc A38 (0.5696, 64.8302) -> (2.6411, 61.8149) centre (5.2326, 65.8145) ccw projected
  arc A39 (16.4257, 62.6549) -> (17.1363, 62.5661) centre (16.7931, 62.7074) ccw projected
  arc A40 (17.1363, 62.5661) -> (18.4601, 59.2911) centre (21.1825, 62.2965) ccw projected
  line L7 (18.4601, 59.2911) -> (13.9877, 60.285) projected
  arc A41 (13.9877, 60.285) -> (16.4257, 62.6549) centre (12.0514, 64.7157) ccw projected
  line L8 (-13.3984, 60.2835) -> (-17.5857, 59.3699) projected
  arc A42 (-17.5857, 59.3699) -> (-16.8326, 62.2884) centre (-20.4564, 61.6671) ccw projected
  arc A43 (-16.8326, 62.2884) -> (-16.1185, 62.6849) centre (-16.5732, 62.6625) ccw projected
  arc A44 (-16.1185, 62.6849) -> (-13.3984, 60.2835) centre (-10.7455, 66.0297) ccw projected
  arc A45 (23.3101, 59.2794) -> (24.6426, 59.0129) centre (24.1153, 59.8411) ccw projected
  arc A46 (24.6426, 59.0129) -> (26.0136, 56.3094) centre (35.6939, 62.9182) ccw projected
  line L9 (26.0136, 56.3094) -> (20.9448, 58.2972) projected
  arc A47 (20.9448, 58.2972) -> (23.3101, 59.2794) centre (20.4128, 62.9176) ccw projected
  line L10 (-20.7071, 58.4563) -> (-25.3892, 56.4769) projected
  arc A48 (-25.3892, 56.4769) -> (-24.4767, 59.0763) centre (-36.9067, 61.9797) ccw projected
  arc A49 (-24.4767, 59.0763) -> (-23.4267, 59.3699) centre (-24.0109, 59.435) ccw projected
  arc A50 (-23.4267, 59.3699) -> (-20.7071, 58.4563) centre (-19.5919, 66.2806) ccw projected
  line L11 (-5.4311, 61.4871) -> (-10.1889, 61.1777) projected
  arc A51 (-10.1889, 61.1777) -> (-8.6844, 63.2278) centre (-11.7929, 63.9318) ccw projected
  arc A52 (-8.6844, 63.2278) -> (-7.2144, 63.2692) centre (-7.9871, 64.5875) ccw projected
  arc A53 (-7.2144, 63.2692) -> (-5.4311, 61.4871) centre (-1.9408, 66.7629) ccw projected
  arc A54 (7.5609, 63.2438) -> (9.2639, 63.034) centre (8.5734, 64.4461) ccw projected
  arc A55 (9.2639, 63.034) -> (11.0061, 61.2788) centre (13.5712, 65.5673) ccw projected
  line L12 (11.0061, 61.2788) -> (5.99, 61.6262) projected
  arc A56 (5.99, 61.6262) -> (7.5609, 63.2438) centre (5.2448, 63.9213) ccw projected
  circle A57 centre (0, 0) radius 46.6203 projected
  arc A58 (-21.8497, 72.7265) -> (-27.5235, 70.7744) centre (0, 0) ccw
  arc A59 (-2.1604, 75.9071) -> (-15.6689, 74.3037) centre (0, 0) ccw
  arc A60 (27.7023, 70.7046) -> (22.0296, 72.6723) centre (0, 0) ccw
  arc A61 (15.8106, 74.2737) -> (2.2894, 75.9033) centre (0, 0) ccw
  constraints: 14 point on circle, 4 centre point, 2 point on line, 1 coincident
extrude "Extrusion10" add sketch "Sketch49" against normal blind 1 contours A1 A2 A3 A59 L0 A4 L1 A5 A6 A7 A8 A9 A10 A0 | A12 A13 A14 A15 A16 A17 A18 A19 A20 L2 A21 L3 A61 A11 | A22 L4 A23 A24 A25 A26 A27 A28 A58 | A30 A31 A32 L5 A33 A60 A34 A35 A29 | L6 A36 A37 A38 | A39 A40 L7 A41 | L8 A42 A43 A44 | A45 A46 L9 A47 | L10 A48 A49 A50 | L11 A51 A52 A53 | A54 A55 L12 A56
sketch "Sketch52" plane through (0, 0, 3) normal (0, 0, 1) x (1, 0, 0)
  line L0 (-0.6206, 16.6817) -> (-5.8652, 21.5583) projected
  line L1 (7.1383, -0.1113) -> (-7.3583, -0.1113) projected
  line L2 (-7.3583, -0.1113) -> (-7.3583, -21.0954) projected
  arc A0 (-13.1155, 18.0871) -> (-7.3583, -21.0954) centre (0, 0) ccw projected
  line L3 (-13.1155, 18.0871) -> (-0.6206, 4.403) projected
  line L4 (-0.6206, 4.403) -> (12.5775, 18.4653) projected
  arc A1 (20.0006, 9.9568) -> (12.5775, 18.4653) centre (0, 0) ccw projected
  line L5 (20.0006, 9.9568) -> (26.5524, 15.0359) projected
  arc A2 (26.5524, 15.0359) -> (18.22, 24.4773) centre (0, 0) ccw projected
  line L6 (18.22, 24.4773) -> (22.0152, 28.521) projected
  arc A3 (27.8194, -22.8954) -> (22.0152, 28.521) centre (0, 0) ccw projected
  line L7 (27.8194, -22.8954) -> (33.5184, -28.2607) projected
  arc A4 (33.5184, -28.2607) -> (21.4165, 38.2555) centre (0, 0) ccw projected
  line L8 (-11.8672, 28.1119) -> (-21.4067, 38.261) projected
  arc A5 (-21.4067, 38.261) -> (-33.3316, -28.4808) centre (0, 0) ccw projected
  line L9 (-33.3316, -28.4808) -> (-27.8194, -22.8954) projected
  arc A6 (-22.3813, 28.2346) -> (-27.8194, -22.8954) centre (0, 0) ccw projected
  line L10 (-22.3813, 28.2346) -> (-18.6516, 24.1501) projected
  arc A7 (-18.6516, 24.1501) -> (-8.045, -29.4345) centre (0, 0) ccw projected
  line L11 (-8.045, -29.4345) -> (-8.045, -36.0294) projected
  line L12 (-8.045, -36.0294) -> (0, -36.0294) projected
  line L13 (0, -36.0294) -> (0, -30.5141) projected
  arc A8 (0, -30.5141) -> (24.0395, -18.7939) centre (0, 0) ccw projected
  line L14 (24.0395, -18.7939) -> (18.3751, -12.7089) projected
  arc A9 (-1.6668, -22.2796) -> (18.3751, -12.7089) centre (0, 0) ccw projected
  line L15 (-1.6668, -22.2796) -> (-1.6668, -15.2832) projected
  line L16 (-1.6668, -15.2832) -> (7.3438, -15.2832) projected
  line L17 (7.3438, -15.2832) -> (7.3438, -10.1842) projected
  line L18 (7.3438, -10.1842) -> (-1.3429, -10.1842) projected
  line L19 (-1.3429, -10.1842) -> (-1.3429, -4.5649) projected
  line L20 (-1.3429, -4.5649) -> (7.1383, -4.5649) projected
  line L21 (7.1383, -4.5649) -> (7.1383, -0.1113) projected
  line L22 (-22.4548, 29.4441) -> (-0.6206, 5.9887)
  line L23 (21.7212, 29.9894) -> (-0.6206, 5.9887)
  arc A10 (26.5524, 15.0359) -> (18.22, 24.4773) centre (0, 0) ccw
  arc A11 (20.0006, 9.9568) -> (12.5775, 18.4653) centre (0, 0) ccw
  arc A12 (20.8059, 10.5811) -> (13.2698, 19.203) centre (0, 0) ccw
  arc A13 (25.7535, 14.4166) -> (17.5311, 23.7433) centre (0, 0) ccw
  arc A14 (4.9662, 21.783) -> (-5.8652, 21.5583) centre (0, 0) ccw
  arc A15 (-13.1155, 18.0871) -> (18.3751, -12.7089) centre (0, 0) ccw
  arc A16 (6.985, 22.2723) -> (-7.8921, 21.9672) centre (0, 0) ccw
  arc A17 (-13.7939, 18.8301) -> (19.072, -13.4575) centre (0, 0) ccw
  arc A18 (12.1128, 26.914) -> (-12.1134, 26.9137) centre (0, 0) ccw
  arc A19 (-17.975, 23.409) -> (23.3493, -18.0524) centre (0, 0) ccw
  arc A20 (11.8672, 28.1119) -> (-11.8672, 28.1119) centre (0, 0) ccw
  arc A21 (-18.6516, 24.1501) -> (24.0395, -18.7939) centre (0, 0) ccw
  line L24 (21.4165, 38.2555) -> (11.8672, 28.1119)
  line L25 (4.9662, 21.783) -> (-0.6206, 16.6817)
  line L26 (-0.6206, 15.3275) -> (6.985, 22.2723)
  line L27 (-0.6206, 15.3275) -> (-7.8921, 21.9672)
  line L28 (12.1128, 26.914) -> (21.6044, 36.9962)
  line L29 (-11.8672, 28.1119) -> (-21.4067, 38.261)
  line L30 (-21.5953, 37.0015) -> (-12.1134, 26.9137)
  line L31 (18.22, 24.4773) -> (22.0152, 28.521)
  line L32 (-0.6206, 4.403) -> (12.5775, 18.4653)
  line L33 (13.2698, 19.203) -> (17.5311, 23.7433)
  line L34 (-18.6516, 24.1501) -> (-22.3813, 28.2346)
  line L35 (-0.6206, 4.403) -> (-13.1155, 18.0871)
  line L36 (-13.7939, 18.8301) -> (-17.975, 23.409)
  arc A22 (-21.5953, 37.0015) -> (-32.6266, -27.7664) centre (0, 0) ccw
  arc A23 (32.7891, -27.5742) -> (21.6044, 36.9962) centre (0, 0) ccw
  arc A24 (-22.4548, 29.4441) -> (-28.5255, -23.6109) centre (0, 0) ccw
  arc A25 (28.549, -23.5824) -> (21.7212, 29.9894) centre (0, 0) ccw
  line L37 (33.5184, -28.2607) -> (32.7891, -27.5742)
  line L38 (28.549, -23.5824) -> (27.8194, -22.8954)
  line L39 (-33.3316, -28.4808) -> (-32.6266, -27.7664)
  line L40 (-28.5255, -23.6109) -> (-27.8194, -22.8954)
  line L41 (-7.045, -35.0294) -> (-7.045, -29.6897)
  line L42 (-7.045, -35.0294) -> (-1, -35.0294)
  line L43 (-1, -30.4977) -> (-1, -35.0294)
  line L44 (-6.3583, -21.4181) -> (-6.3583, -1.1113)
  line L45 (-6.3583, -1.1113) -> (6.1383, -1.1113)
  line L46 (6.1383, -3.5649) -> (6.1383, -1.1113)
  line L47 (6.1383, -3.5649) -> (-2.3429, -3.5649)
  line L48 (-2.3429, -11.1842) -> (-2.3429, -3.5649)
  line L49 (6.3438, -11.1842) -> (-2.3429, -11.1842)
  line L50 (6.3438, -14.2832) -> (6.3438, -11.1842)
  line L51 (-2.6668, -14.2832) -> (6.3438, -14.2832)
  line L52 (-2.6668, -22.1822) -> (-2.6668, -14.2832)
  point P0 (11.1256, 18.6071)
  constraints: 69 end point, 38 point on circle, 16 centre point, 13 point on line, 8 collinear, 5 coincident, 5 parallel, 3 perpendicular
extrude "Extrusion12" cut sketch "Sketch52" against normal blind 0.01 contours L21 L20 L19 L18 L17 L16 L15 A15 L52 L51 L50 L49 L48 L47 L46 L45 L44 L2 L1 | A15 A9 L14 A17 L36 A19 A8 A21 A7 L10 A6 L9 A24 L22 L23 A25 L7 A3 L6 A2 L5 A13 L33 A12 A1 L4 L3 A0 | L13 L12 L11 A21 L41 L42 L43 | A23 L28 A18 L30 A22 L9 A5 L8 A20 L24 A4 L7 | L26 L27 A16
sketch "Sketch53" plane through (0, 0, 3) normal (0, 0, 1) x (1, 0, 0)
  circle A0 centre (0, 0) radius 46.6203 projected
  circle A1 centre (0, 0) radius 51 projected
  circle A2 centre (0, 0) radius 50
  circle A3 centre (0, 0) radius 47.6203
  constraints: 2 centre point, 2 coincident
extrude "Extrusion13" cut sketch "Sketch53" against normal blind 0.01
body "Solid1"
